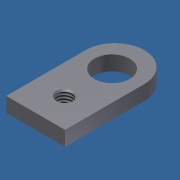
# Autodesk Inventor part: SUPORTE DO EIXO TRASEIRO(51)
Saved by Autodesk Inventor 2012 SP2 (Build 160219200, 219)
## iProperties
Created: 2012-07-23
Part Number: SUPORTE DO EIXO TRASEIRO(51)
Material: Carbon Steel
Document SubType Name: Modeling
Designer: bruno.silveira
Mass: 22.2001 g
Surface Area: 19.144 cm^2
Volume: 2.82085 cm^3
Density: 7.87 g/cm^3
Author: bruno.silveira
Autodesk Inventor part; units mm, degrees
ref_plane "YZ Plane" through (0, 0, 0) normal (1, 0, 0) x (0, 1, 0)
ref_plane "XZ Plane" through (0, 0, 0) normal (0, 1, 0) x (-1, 0, 0)
ref_plane "XY Plane" through (0, 0, 0) normal (0, 0, 1) x (1, 0, 0)
sketch "Sketch1" plane through (0, 0, 0) normal (0, 0, 1) x (1, 0, 0)
  line L0 (0, 0) -> (20, 0)
  line L1 (20, 0) -> (20, 37)
  line L2 (20, 37) -> (0, 37)
  line L3 (0, 37) -> (0, 0)
  dimension "d0" = 20
  dimension "d1" = 37
  constraints: 8 end point, 2 parallel, 1 horizontal, 1 perpendicular
  measures "d0" distance of L1.end L2.end
  measures "d1" distance of L2.end L0.start
extrude "Extrusion1" add sketch "Sketch1" along normal blind 5
sketch "Sketch2" plane through (0, 0, 5) normal (0, 0, 1) x (1, 0, 0)
  line L0 (20, 0) -> (0, 0) projected
  line L1 (20, 37) -> (20, 0) projected
  point P0 (10, 26)
  dimension "d4" = 26
  dimension "d5" = 10
  measures "d4" distance from line of L0 point (10, 26)
  measures "d5" distance from line of L1 point (10, 26)
hole "Hole1" at (10, 26, 5) direction (0, 0, -1) diameter 12 depth 5 tip angle 118
fillet "Fillet1" radius 10 2 edges at (20, 37, 2.5) (0, 37, 2.5)
sketch "Sketch3" plane through (0, 0, 5) normal (0, 0, 1) x (1, 0, 0)
  line L0 (0, 0) -> (0, 27) projected
  line L1 (20, 0) -> (0, 0) projected
  point P0 (10, 10)
  dimension "d14" = 10
  dimension "d15" = 10
  measures "d14" distance from line of L1 point (10, 10)
  measures "d15" distance from line of L0 point (10, 10)
hole "Hole2" at (10, 10, 5) direction (0, 0, -1) diameter 4.917 depth 6 tip angle 118 thread size "M6x1" class "6H" standard "ANSI Metric M Profile"
chamfer "Chamfer1" distance 0.5 angle 45 2 edges at (10, 12.4585, 5) (10, 12.4585, 0)
body "Solid1"
